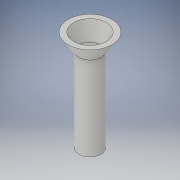
# Autodesk Inventor part: Part2
Saved by Autodesk Inventor 2018 (Build 220112000, 112)
## iProperties
Created: 2018-10-16
Part Number: Part2
Material: Generic
Document SubType Name: Modeling
Designer: Abhay
Density: 1 g/cm^3
Appearance: Default
Author: Abhay
Autodesk Inventor part; units mm, degrees
ref_plane "YZ Plane" through (0, 0, 0) normal (1, 0, 0) x (0, 1, 0)
ref_plane "XZ Plane" through (0, 0, 0) normal (0, 1, 0) x (-1, 0, 0)
ref_plane "XY Plane" through (0, 0, 0) normal (0, 0, 1) x (1, 0, 0)
sketch "Sketch1" plane through (0, 0, 0) normal (0, 0, 1) x (1, 0, 0)
  line L0 (2.0002, 0) -> (1.009, -1.5087)
  line L1 (1.009, -1.5087) -> (1.009, -9.178)
  line L2 (2.0002, 0) -> (0, 0)
  line L3 (0, 0) -> (0, -9.178)
  line L4 (0, -9.178) -> (1.009, -9.178)
  constraints: 10 end point, 2 perpendicular, 1 horizontal
revolve "Revolution1" add sketch "Sketch1" angle 360 about axis through (0, 0, 0) along (0, -1, 0)
sketch "Sketch2" plane through (0, 0, 0) normal (0, 1, 0) x (1, 0, 0)
  circle A0 centre (0, 0) radius 1.4988
  constraints: 1 centre point, 1 coincident
loft "Loft1" cut profiles "Sketch2" section 2 edges at (-1.009, -1.5087, 0)
body "Solid1"
